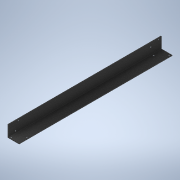
# Autodesk Inventor part: angleline-cross-400
Saved by Autodesk Inventor 2020.4 (Build 244396000, 396)
## iProperties
Created: 2021-02-28
Part Number: angleline-cross-400
Material: Steel
Document SubType Name: Modeling
Designer: AOB
Mass: 472.246 g
Surface Area: 778.462 cm^2
Volume: 60.1588 cm^3
Density: 7.85 g/cm^3
Appearance: Black Cast
Author: AOB
Autodesk Inventor part; units mm, degrees
ref_plane "YZ Plane" through (0, 0, 0) normal (1, 0, 0) x (0, 1, 0)
ref_plane "XZ Plane" through (0, 0, 0) normal (0, 1, 0) x (-1, 0, 0)
ref_plane "XY Plane" through (0, 0, 0) normal (0, 0, 1) x (1, 0, 0)
sketch "Sketch1" plane through (0, 0, 0) normal (0, 0, 1) x (1, 0, 0)
  line L0 (0, 0) -> (0, -38.1)
  line L1 (0, -38.1) -> (38.1, -38.1)
  line L2 (38.1, -38.1) -> (38.1, -36.5125)
  line L3 (38.1, -36.5125) -> (1.5875, -36.5125)
  line L4 (1.5875, -36.5125) -> (1.5875, 0)
  line L5 (1.5875, 0) -> (0, 0)
  dimension "d0" = 1.5875
  dimension "d1" = 1.5875
  dimension "d2" = 38.1
  dimension "d3" = 38.1
  constraints: 12 end point, 5 perpendicular, 1 vertical
  measures "d0" distance of L1.end L2.end
  measures "d1" distance of L4.end L0.start
  measures "d2" distance of L0.start L0.end
  measures "d3" distance of L0.end L1.end
extrude "Extrusion1" add sketch "Sketch1" along normal blind 510
sketch "Sketch2" plane through (0, -38.1, 0) normal (0, -1, 0) x (1, 0, 0)
  line L0 (1.5875, 0.1232) -> (38.1, 0.1232)
  line L1 (38.1, 0.1232) -> (38.1, 36.5227)
  line L2 (38.1, 36.5227) -> (1.5875, 36.5227)
  line L3 (1.5875, 36.5227) -> (1.5875, 0.1232)
  line L4 (1.5875, 473.4875) -> (38.1, 473.4875)
  line L5 (38.1, 473.4875) -> (38.1, 510)
  line L6 (38.1, 510) -> (1.5875, 510)
  line L7 (1.5875, 510) -> (1.5875, 473.4875)
  line L8 (0, 0) -> (0, 37)
  line L9 (0, 365.3234) -> (0, 400)
  line L10 (0, 0) -> (0, 510) projected
  line L11 (0, 510) -> (38.1, 510) projected
  line L12 (1.5875, 0) -> (1.5875, 510) construction
  line L13 (1.5875, 36.5227) -> (7.1068, 31.2689)
  line L14 (38.1, 473.4875) -> (1.5875, 510) construction
  line L15 (38.1, 473.4875) -> (32.7118, 478.8757)
  line L16 (1.5875, 510) -> (6.9757, 504.6118)
  line L17 (0, 0) -> (38.1, 0) projected
  line L18 (38.1, 0) -> (38.1, 36.5227)
  line L19 (38.1, 0) -> (38.1, 510) projected
  line L20 (1.5875, 36.5227) -> (1.5875, 0)
  line L21 (38.1, 0) -> (1.5875, 36.5227) construction
  line L22 (38.1, 0) -> (32.6514, 5.4501)
  dimension "d6" = 36.5227
  dimension "d38" = 36.5125
  dimension "d39" = 36.5125
  dimension "d88" = 7.62
  dimension "d89" = 7.62
  dimension "d90" = 7.62
  dimension "d98" = 7.62
  constraints: 36 end point, 7 point on line, 5 parallel, 2 horizontal, 2 perpendicular, 1 other
  measures "d6" distance of L2.end L12.start
  measures "d38" distance of L1.end L2.end
  measures "d39" distance of L6.end L4.start
  measures "d88" distance of L2.end L13.end
  measures "d89" distance of L4.end L15.end
  measures "d90" distance of L6.end L16.end
  measures "d98" distance of L0.end L22.end
sketch "Sketch3" plane through (0, -38.1, 0) normal (-1, 0, 0) x (0, 0, 1)
  line L0 (3.175, 1.5875) -> (39.6875, 1.5875)
  line L1 (39.6875, 1.5875) -> (39.6875, 38.1)
  line L2 (470.3125, 38.1) -> (470.3125, 1.5875)
  line L3 (470.3125, 1.5875) -> (506.825, 1.5875)
  line L4 (510, 38.1) -> (470.3125, 38.1)
  line L5 (0, 1.5875) -> (0, 38.1) projected
  line L6 (470.3125, 38.1) -> (476.0031, 33.0323)
  line L7 (0, 38.1) -> (510, 38.1) projected
  line L8 (39.6875, 38.1) -> (3.175, 38.1)
  line L9 (400, 0) -> (400, 1.5875)
  line L10 (506.825, 6.9518) -> (484.6, 6.9518) construction
  line L11 (0, 1.5875) -> (510, 1.5875) projected
  line L12 (484.6, 1.5875) -> (484.6, 6.9518)
  line L13 (506.825, 1.5875) -> (506.825, 38.1)
  line L14 (3.175, 1.5875) -> (3.175, 38.1)
  line L15 (34.2993, 1.5875) -> (34.2993, 23.8125)
  line L16 (36.5125, 1.5875) -> (39.6875, 1.5875)
  point P0 (34.2993, 6.9757)
  point P1 (8.5632, 32.7118)
  dimension "d53" = 36.5125
  dimension "d55" = 36.5125
  dimension "d109" = 7.62
  dimension "d122" = 36.5125
  dimension "d123" = 22.225
  dimension "d127" = 22.225
  dimension "d135" = 3.175
  dimension "d136" = 36.5125
  dimension "d137" = 3.175
  constraints: 28 end point, 4 vertical, 2 perpendicular, 2 point on line, 1 collinear, 1 parallel, 5 other
  measures "d53" distance of L0.end L1.end
  measures "d55" distance of L4.start point (510, 1.588)
  measures "d109" distance of L2.start L6.end
  measures "d122" distance of L3.end L2.end
  measures "d123" distance of L10.start L10.end
  measures "d127" distance of L15.start L15.end
  measures "d135" distance of L16.start L16.end
  measures "d136" distance of L1.end L8.end
  measures "d137" distance of point (510, 1.588) L3.end
hole "Hole8" at (32.7118, -38.1, 478.8757) at (6.9757, -38.1, 504.6118) at (7.1068, -38.1, 31.2689) direction (0, 1, 0) diameter 5 end through all
hole "Hole9" at (32.6514, -38.1, 5.4501) direction (0, 1, 0) diameter 5 end through all
hole "Hole11" at (0, -31.1482, 484.6) at (0, -5.0677, 476.0031) at (0, -14.2875, 34.2993) at (0, -5.3882, 8.5632) direction (1, 0, 0) diameter 5 end through all
equation "\"d39\" = d38"
equation "\"d55\" = d53"
body "Solid1"
